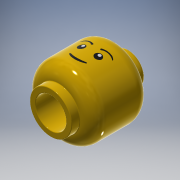
# Autodesk Inventor part: Cabeza lego
Saved by Autodesk Inventor 2017 (Build 210142000, 142)
## iProperties
Created: 2017-06-23
Part Number: Cabeza lego
Material: Plástico ABS
Document SubType Name: Modeling
Designer: H. Valenzuela B.
Density: 1.06 g/cm^3
Appearance: Suave - Blanco
Author: H. Valenzuela B.
Autodesk Inventor part; units mm, degrees
ref_plane "YZ Plane" through (0, 0, 0) normal (1, 0, 0) x (0, 1, 0)
ref_plane "XZ Plane" through (0, 0, 0) normal (0, 1, 0) x (-1, 0, 0)
sketch "Boceto1" plane through (0, 0, 0) normal (0, 0, 1) x (1, 0, 0)
  line L0 (-6.6171, 0) -> (1.1028, 0) construction
  line L1 (0, -2.3407) -> (0, 14.0443) construction
  line L2 (-1.5, 11.6) -> (-1.5, 8.7)
  line L3 (-1.5, 8.7) -> (-2.25, 8.7)
  line L4 (-2.25, 8.7) -> (-2.25, 0)
  line L5 (-3.1, 0) -> (-2.25, 0)
  line L6 (-3.1, 0) -> (-3.1, 1.2)
  line L7 (-3.1, 1.2) -> (-3.1, 1.2)
  line L8 (-5.1, 3.2) -> (-5.1, 7.8)
  line L9 (-3.1, 9.8) -> (-2.45, 9.8)
  line L10 (-2.45, 9.8) -> (-2.45, 11.1)
  line L11 (-1.95, 11.6) -> (-1.5, 11.6)
  arc A0 (-3.1, 9.8) -> (-5.1, 7.8) centre (-3.1, 7.8) ccw
  arc A1 (-5.1, 3.2) -> (-3.1, 1.2) centre (-3.1, 3.2) ccw
  arc A2 (-1.95, 11.6) -> (-2.45, 11.1) centre (-1.95, 11.1) ccw
  point P0 (0, 0)
  dimension "d0" = 3
  dimension "d1" = 4.9
  dimension "d2" = 10.2
  dimension "d18" = 1.8
  dimension "d19" = 8.6
  dimension "d20" = 2
  dimension "d34" = 0
  dimension "d35" = 1.2
  dimension "d46" = 0.5
  dimension "d50" = 8.7
  dimension "d51" = 4.5
  constraints: 20 end point, 7 perpendicular, 6 point on circle, 6 tangent, 3 centre point, 2 point on line, 2 vertical, 1 collinear, 1 equal radius
  measures "d0" diameter of L2 L1
  measures "d1" diameter of L10 L1
  measures "d2" diameter of L8 L1
  measures "d18" distance between parallel lines of L9 L11
  measures "d19" distance between parallel lines of L7 L9
  measures "d20" radius of A0
  measures "d34" distance of L6.end L7.end
  measures "d35" distance of L5.start L6.end
  measures "d46" radius of A2
  measures "d50" distance between parallel lines of L0 L3
  measures "d51" diameter of L4 L1
revolve "Revolución1" add sketch "Boceto1" angle 360 about axis through (0, -10, 0) along (0, 1, 0)
fillet "Empalme1" radius 0.1 5 edges at (2.45, 9.8, 0) (3.1, 1.2, 0) (2.25, 0, 0) (1.5, 11.6, 0) (3.1, 0, 0)
ref_plane "Plano de trabajo1" through (0, 0, 6) normal (0, 0, 1) x (1, 0, 0)
sketch "Boceto2" plane through (0, 0, 6) normal (0, 0, 1) x (1, 0, 0)
  arc A0 (-1.9324, 7.1182) -> (-2.4885, 6.8178) centre (-1.7952, 6.1994) ccw
  arc A1 (-0.6302, 6.9298) -> (-1.9324, 7.1182) centre (-1.5948, 4.8576) ccw
  arc A2 (-0.5499, 6.8163) -> (-0.6302, 6.9298) centre (-0.6893, 6.8029) ccw
  arc A3 (-0.7876, 6.7032) -> (-0.5499, 6.8163) centre (-0.6893, 6.8029) ccw
  arc A4 (-0.7876, 6.7032) -> (-1.0167, 6.8525) centre (-1.268, 6.2167) ccw
  arc A5 (-2.4885, 6.8178) -> (-2.4257, 6.7415) centre (-2.4512, 6.7845) ccw
  circle A6 centre (-1.2506, 5.79) radius 0.5209
  circle A7 centre (-1.2228, 6.0055) radius 0.2278
  line L0 (0, -2.32) -> (0, 13.92) projected
  line L1 (-6, 12.192) -> (6, 12.192) construction
  line L2 (6, 12.192) -> (6, 0.792) construction
  line L3 (6, 0.792) -> (-6, 0.792) construction
  line L4 (-6, 0.792) -> (-6, 12.192) construction
  arc A8 (-1.0167, 6.8525) -> (-2.4257, 6.7415) centre (-1.6077, 5.3568) ccw
  arc A9 (-1.1964, 4.1443) -> (1.1454, 4.1336) centre (-0.0143, 6.6103) ccw
  arc A10 (1.2463, 3.9708) -> (1.1454, 4.1336) centre (1.1863, 4.0463) ccw
  arc A11 (-1.1964, 4.1443) -> (-1.2656, 3.9659) centre (-1.2037, 4.0445) ccw
  arc A12 (-1.2656, 3.9659) -> (1.2463, 3.9708) centre (-0.0127, 5.554) ccw
  point P0 (0, 0)
  dimension "d93" = 0.05
  dimension "d94" = 0.14
  dimension "d106" = 12
  dimension "d118" = 6.1994
  dimension "d119" = 0.6893
  dimension "d120" = 2.4512
  dimension "d121" = 6.8029
  dimension "d122" = 6.7845
  dimension "d123" = 2.2857
  dimension "d124" = 0.929
  constraints: 23 point on circle, 13 centre point, 9 tangent, 1 concentric, 3 other
  measures "d93" radius of A5
  measures "d94" radius of A3
  measures "d106" distance of L1.start L1.end
  measures "d118" vertical distance of point (0, 0) A0.centre
  measures "d119" distance from line of L0 A3.centre
  measures "d120" distance from line of L0 A5.centre
  measures "d121" vertical distance of A3.centre point (0, 0)
  measures "d122" vertical distance of point (0, 0) A5.centre
  measures "d123" radius of A1
  measures "d124" radius of A0
emboss "Repujado1" sketch "Boceto2" operation cut depth 0.01 direction (0, 0, 1) wrap yes faces at (-5.034, 4.7333, -0.8181) contours A1 A2 A3 A4 A8 A5 A0 | A6
emboss "Repujado2" sketch "Boceto2" operation cut depth 0.01 direction (0, 0, 1) wrap yes faces at (-3.3881, 5.9176, 3.8119) contours A12 A11 A9 L0 | L0 A9 A10 A12
mirror "Simetría1" about plane through (0, 0, 0) normal (1, 0, 0) of "Repujado1"
